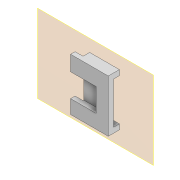
# Autodesk Inventor part: Anglerfish_Cameraspacer
Saved by Autodesk Inventor 2022 (Build 260153000, 153)
## iProperties
Created: 2022-08-19
Part Number: Anglerfish_Cameraspacer
Material: Generisch
Document SubType Name: Modeling
Designer: UC2
Density: 1 g/cm^3
Appearance: Vorgabe
Author: UC2
Autodesk Inventor part; units mm, degrees
ref_plane "YZ Plane" through (0, 0, 0) normal (1, 0, 0) x (0, 1, 0)
ref_plane "XZ Plane" through (0, 0, 0) normal (0, 1, 0) x (-1, 0, 0)
ref_plane "XY Plane" through (0, 0, 0) normal (0, 0, 1) x (1, 0, 0)
ref_plane "Arbeitsebene1" through (0, 0, 0) normal (0, 0, 1) x (1, 0, 0)
sketch "Skizze1" plane through (0, 0, 0) normal (0, 0, 1) x (1, 0, 0)
  circle A0 centre (-0.0001, 0.0021) radius 3 projected
  circle A1 centre (11, 0) radius 2.566 projected
  circle A2 centre (-9.5, -11) radius 1.352 projected
  arc A3 (19, -13.5) -> (20, -12.5) centre (19, -12.5) ccw projected
  line L0 (20, -12.5) -> (20, 12.5) projected
  arc A4 (20, 12.5) -> (19, 13.5) centre (19, 12.5) ccw projected
  line L1 (19, 13.5) -> (-19, 13.5) projected
  arc A5 (-19, 13.5) -> (-20, 12.5) centre (-19, 12.5) ccw projected
  line L2 (-20, 12.5) -> (-20, -12.5) projected
  arc A6 (-20, -12.5) -> (-19, -13.5) centre (-19, -12.5) ccw projected
  line L3 (-19, -13.5) -> (19, -13.5) projected
  line L4 (18.6579, -7.132) -> (11.0758, -7.132) projected
  line L5 (18.6579, -7.132) -> (18.6579, 2.268) projected
  line L6 (18.6579, 2.268) -> (19.6579, 4.268) projected
  line L7 (19.6579, 4.268) -> (19.6579, 7.668) projected
  line L8 (18.0704, 7.668) -> (19.6579, 7.668) projected
  line L9 (18.0704, 7.668) -> (18.0704, 6.818) projected
  line L10 (18.0704, 6.818) -> (13.4704, 6.818) projected
  line L11 (13.4704, 6.818) -> (13.4704, 5.418) projected
  line L12 (13.4704, 5.418) -> (14.8704, 5.418) projected
  line L13 (14.8704, 5.418) -> (15.4704, 6.018) projected
  line L14 (15.4704, 6.018) -> (18.0704, 6.018) projected
  line L15 (18.0704, 6.018) -> (18.0704, 5.768) projected
  line L16 (18.0704, 5.768) -> (15.5704, 5.768) projected
  line L17 (15.5704, 5.768) -> (15.0704, 5.268) projected
  line L18 (15.0704, 5.268) -> (13.0704, 5.268) projected
  line L19 (13.0704, 5.268) -> (13.0704, 7.668) projected
  line L20 (6.4079, 7.668) -> (13.0704, 7.668) projected
  line L21 (6.4079, 7.668) -> (6.4079, 6.468) projected
  line L22 (4.7579, 6.468) -> (6.4079, 6.468) projected
  line L23 (4.7579, -7.132) -> (4.7579, 6.468) projected
  line L24 (5.4458, -7.132) -> (4.7579, -7.132) projected
  line L25 (5.4458, -7.132) -> (5.4458, -6.382) projected
  line L26 (5.4458, -6.382) -> (11.0758, -6.382) projected
  line L27 (11.0758, -6.382) -> (11.0758, -7.132) projected
  line L28 (9.0327, 10.168) -> (-5.2421, 10.168)
  line L29 (-5.2421, 10.168) -> (-5.2421, 8.168)
  line L30 (-5.2421, 8.168) -> (9.0327, 8.168)
  line L31 (9.0327, 8.168) -> (9.0327, 10.168)
  line L32 (-5.2421, 8.168) -> (4.7579, 8.168)
  line L33 (4.7579, 8.168) -> (4.7579, -9.632)
  line L34 (4.7579, -9.632) -> (-5.2421, -9.632)
  line L35 (-5.2421, -9.632) -> (-5.2421, 8.168)
  line L36 (4.7579, -9.632) -> (9.0327, -9.632)
  line L37 (9.0327, -9.632) -> (9.0327, -7.632)
  line L38 (9.0327, -7.632) -> (4.7579, -7.632)
  line L39 (4.7579, -7.632) -> (4.7579, -9.632)
  point P0 (0, 0)
  point P1 (4.7579, 8.168)
  dimension "d0" = 0
  dimension "d1" = 0.5
  dimension "d2" = 0.5
  dimension "d3" = 2
  dimension "d4" = 2
  dimension "d5" = 10
  constraints: 24 end point, 6 parallel, 3 horizontal, 3 perpendicular, 1 point on line
  measures "d0" distance between parallel lines of L23 L33
  measures "d1" distance between parallel lines of L20 L30
  measures "d2" distance from line of L38 L24.start
  measures "d3" distance between parallel lines of L38 L36
  measures "d4" distance between parallel lines of L30 L28
  measures "d5" distance between parallel lines of L35 L33
ref_plane "Arbeitsebene2" through (4.7579, -7.132, 2.2) normal (0, 0, 1) x (1, 0, 0)
extrude "Extrusion1" add sketch "Skizze1" along normal up to surface (2.2 mm away) contours A0 | L33 L34 L35 L30 L23 | L38 L37 L36 L33 | L30 L29 L28 L31
sketch "Skizze2" plane through (-5.2421, 10.168, 2.2) normal (0, 0, 1) x (1, 0, 0)
  line L0 (0, 0) -> (14.2747, 0) projected
  line L1 (0, -19.8) -> (0, 0) projected
  line L2 (14.2747, -19.8) -> (0, -19.8) projected
  line L3 (14.2747, -17.8) -> (14.2747, -19.8) projected
  line L4 (10, -17.8) -> (14.2747, -17.8) projected
  line L5 (10, -2) -> (10, -17.8) projected
  line L6 (14.2747, -2) -> (10, -2) projected
  line L7 (14.2747, 0) -> (14.2747, -2) projected
  line L8 (14.2747, 0) -> (0, 0) projected
  line L9 (14.2747, 0) -> (0, 0)
  line L10 (0, 0) -> (0, -19.8)
  line L11 (0, -19.8) -> (14.2747, -19.8)
  line L12 (14.2747, -19.8) -> (14.2747, 0)
  line L13 (9.6421, -14.568) -> (0.8421, -14.568)
  line L14 (0.8421, -14.568) -> (0.8421, -5.768)
  line L15 (0.8421, -5.768) -> (9.6421, -5.768)
  line L16 (9.6421, -5.768) -> (9.6421, -14.568)
  line L17 (9.6421, -14.568) -> (0.8421, -5.768) construction
  line L18 (0.8421, -14.568) -> (9.6421, -5.768) construction
  line L19 (0, 0) -> (0, -19.8) projected
  line L20 (0.8421, -5.768) -> (0, -5.768)
  line L21 (0, -5.768) -> (0, -14.568)
  line L22 (0, -14.568) -> (0.8421, -14.568)
  line L23 (0.8421, -14.568) -> (0.8421, -5.768)
  point P0 (5.2421, -10.168)
  point P1 (0, -5.768)
  point P2 (0.8421, -14.568)
  point P3 (14.2747, -17.8)
  point P4 (14.2747, -2)
  dimension "d8" = 8.8
  dimension "d9" = 8.8
  constraints: 28 end point, 6 parallel, 3 horizontal, 3 perpendicular, 2 midpoint, 1 point on line
  measures "d8" distance of L14.end L15.end
  measures "d9" distance of L13.end L14.end
extrude "Extrusion2" add sketch "Skizze2" along normal blind 2 contours L0 L7 L6 L5 L4 L3 L2 L1 L22 L13 L16 L15 L20 | L12 L4 L5 L6
sketch "Skizze3" plane through (0, 0, 0) normal (0, 0, -1) x (-1, 0, 0)
  line L0 (5.2421, 10.168) -> (5.2421, -9.632) projected
  line L1 (-9.0327, 10.168) -> (5.2421, 10.168) projected
  line L2 (-9.0327, 8.168) -> (-9.0327, 10.168) projected
  line L3 (-4.7579, 8.168) -> (-9.0327, 8.168) projected
  line L4 (-4.7579, -7.632) -> (-4.7579, 8.168) projected
  line L5 (-9.0327, -7.632) -> (-4.7579, -7.632) projected
  line L6 (-9.0327, -9.632) -> (-9.0327, -7.632) projected
  line L7 (5.2421, -9.632) -> (-9.0327, -9.632) projected
  line L8 (2.2421, -9.8367) -> (9.0217, -9.8367)
  line L9 (9.0217, -9.8367) -> (9.0217, 10.4786)
  line L10 (9.0217, 10.4786) -> (2.2421, 10.4786)
  line L11 (2.2421, 10.4786) -> (2.2421, -9.8367)
  line L12 (2.2421, -9.8367) -> (9.0217, 10.4786) construction
  line L13 (9.0217, -9.8367) -> (2.2421, 10.4786) construction
  point P0 (0, 0)
  point P1 (5.6319, 0.321)
  dimension "d12" = 3
  constraints: 12 end point, 2 midpoint, 2 parallel, 1 horizontal, 1 perpendicular
  measures "d12" distance between parallel lines of L11 L0
extrude "Extrusion3" cut sketch "Skizze3" against normal blind 2.5 contours L1 L11 L10 L9 L8 L7 L0 | L0 L7 L11 L1
equation "\"d6\" = d2"
